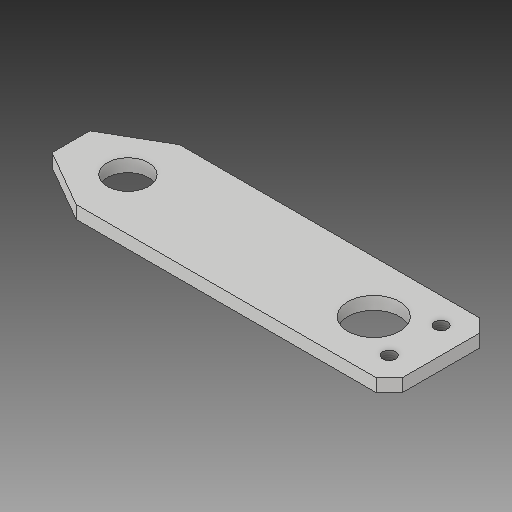
# Autodesk Inventor part: bočnice
Saved by Autodesk Inventor 2019 (Build 230136000, 136)
## iProperties
Created: 2018-11-24
Part Number: bočnice
Material: Generic
Document SubType Name: Modeling
Designer: Radek
Density: 1 g/cm^3
Appearance: Default
Author: Radek
Autodesk Inventor part; units mm, degrees
ref_plane "YZ Plane" through (0, 0, 0) normal (1, 0, 0) x (0, 1, 0)
ref_plane "XZ Plane" through (0, 0, 0) normal (0, 1, 0) x (-1, 0, 0)
ref_plane "XY Plane" through (0, 0, 0) normal (0, 0, 1) x (1, 0, 0)
sketch "Náčrt1" plane through (0, 0, 0) normal (0, 1, 0) x (-1, 0, 0)
  line L0 (0, 0) -> (116, 0)
  line L1 (116, -40) -> (0, -40)
  circle A0 centre (21, -20) radius 10
  line L2 (116, 0) -> (138, -12.7017)
  line L3 (138, -12.7017) -> (138, -27.2983)
  line L4 (138, -27.2983) -> (116, -40)
  line L5 (0, 0) -> (-5, -5)
  line L6 (-5, -5) -> (-5, -35)
  line L7 (-5, -35) -> (0, -40)
  circle A1 centre (116, -20) radius 8
  circle A2 centre (5, -30) radius 2.5
  circle A3 centre (5, -10) radius 2.5
  dimension "d0" = 5
  dimension "d1" = 5
  dimension "d2" = 5
  dimension "d3" = 143
  dimension "d4" = 16
  dimension "d5" = 20
  dimension "d6" = 40
  dimension "d7" = 20
  dimension "d8" = 26
  dimension "d9" = 30
  dimension "d10" = 95
  dimension "d11" = 121
  dimension "d13" = 30
  dimension "d14" = 20
  dimension "d15" = 5
  dimension "d16" = 5
  dimension "d17" = 10
  dimension "d18" = 10
  dimension "d19" = 10
  dimension "d20" = 10
  constraints: 16 end point, 4 centre point, 2 vertical, 1 equal length, 1 horizontal, 1 parallel, 1 perpendicular
  measures "d0" horizontal distance of L6.end L1.end
  measures "d1" horizontal distance of L6.end L1.end
  measures "d2" horizontal distance of L0.start L5.end
  measures "d3" distance between parallel lines of L6 L3
  measures "d4" diameter of A1
  measures "d5" distance from line of L1 A1.centre
  measures "d6" distance between parallel lines of L1 L0
  measures "d7" distance from line of L1 A0.centre
  measures "d8" distance from line of L6 A0.centre
  measures "d9" angle of L1 L4
  measures "d10" distance of A0.centre A1.centre
  measures "d11" distance from line of L6 L1.start
  measures "d13" angle of L0 L2
  measures "d14" diameter of A0
  measures "d15" diameter of A2
  measures "d16" diameter of A3
  measures "d17" distance from line of L6 A2.centre
  measures "d18" distance from line of L1 A2.centre
  measures "d19" distance from line of L6 A3.centre
  measures "d20" distance from line of L0 A3.centre
extrude "Vysunutí1" add sketch "Náčrt1" along normal blind 5
thread "Závit1" size "M5x0.8" class "6H" standard "ANSI Metric M Profile" full length
thread "Závit2" size "M5x0.8" class "6H" standard "ANSI Metric M Profile" full length
equation "\"d11\" = d10 + d8"
equation "\"d13\" = d9"
